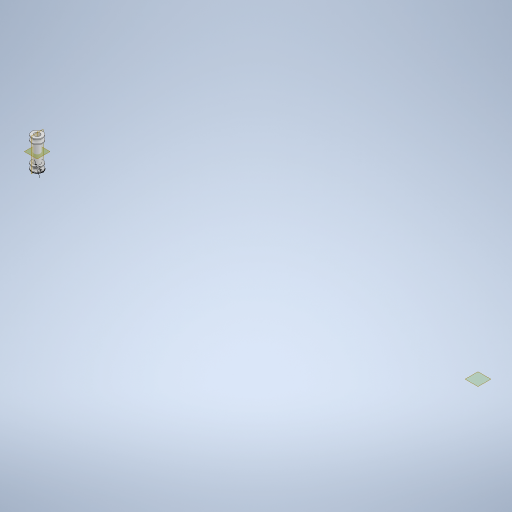
# Autodesk Inventor part: 코일감는원통1
Saved by Autodesk Inventor 2023 (Build 270158000, 158)
## iProperties
Created: 2023-04-25
Part Number: 코일감는원통1
Material: 일반
Document SubType Name: Modeling
Designer: rlatk
Density: 1 g/cm^3
Appearance: 기본값
Author: rlatk
Autodesk Inventor part; units mm, degrees
ref_plane "XZ Plane" through (0, 0, 0) normal (0, 1, 0) x (-1, 0, 0)
ref_plane "XY Plane" through (0, 0, 0) normal (0, 0, 1) x (1, 0, 0)
sketch "스케치1" plane through (0, 0, 0) normal (0, 1, 0) x (-1, 0, 0)
  circle A0 centre (0, 0) radius 5.1
  circle A1 centre (0, 0) radius 6.1
  circle A2 centre (0, 0) radius 10.1
  dimension "d0" = 10.2
  dimension "d1" = 1
  dimension "d2" = 5
  constraints: 3 centre point, 1 coincident
  measures "d0" diameter of A0
  measures "d1" radial gap between concentric circles of A0 A1
  measures "d2" radial gap between concentric circles of A0 A2
extrude "돌출1" add sketch "스케치1" along normal blind 56 contours A1
extrude "돌출2" add sketch "스케치1" along normal blind 10 contours A2
ref_plane "작업 평면1" through (0, 0, 0) normal (0, -1, 0) x (1, 0, 0)
ref_plane "작업 평면2" through (0, 28, 0) normal (0, -1, 0) x (1, 0, 0)
mirror "미러1" about plane through (0, 28, 0) normal (0, -1, 0) of "돌출2"
sketch "스케치2" plane through (0, 0, 0) normal (1, 0, 0) x (0, 1, 0)
  point P0 (0, 0)
sketch "스케치3" plane through (0, 0, 0) normal (1, 0, 0) x (0, 1, 0)
  line L0 (56, -10.1) -> (56, 10.1) projected
  line L1 (46, -10.1) -> (56, -10.1) projected
  line L2 (56, -10.1) -> (46, -10.1)
  arc A0 (54.5, -10.1) -> (47.5, -10.1) centre (51, -12.0365) ccw
  line L3 (-11.2, 0) -> (67.2, 0) projected
  point P0 (0, 0)
  point P1 (47.5, -10.1)
  dimension "d9" = 4
  dimension "d10" = 1.5
  dimension "d11" = 1.5
  constraints: 2 end point, 2 point on circle, 2 point on line, 1 centre point, 1 collinear
  measures "d9" radius of A0
  measures "d10" distance of L0.start A0.start
  measures "d11" distance of L1.start A0.end
revolve "회전1" cut sketch "스케치3" angle 360 about axis through (0, -10, 0) along (0, 1, 0)
mirror "미러4" about plane through (0, 28, 0) normal (0, -1, 0) of "회전1"
ref_plane "작업 평면3" through (0, 28, 0) normal (0, -1, 0) x (1, 0, 0)
